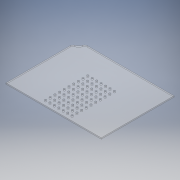
# Autodesk Inventor part: Plaque inferieur
Saved by Autodesk Inventor 2017 (Build 210142000, 142)
## iProperties
Company: FABLAB Frenchmakers
Part Number: Plaque inferieur
Project: 1400-PopCorn Machine
Material: Plastique PMMA
Catalog Web Link: http://www.frenchmakers.com/
Document SubType Name: Modeling
Designer: FABLAB Frenchmakers
Density: 1.188 g/cm^3
Appearance: Polycarbonate - Transparent
Stock Number: 1400-04-01
Author: Adrien MARY
Autodesk Inventor part; units mm, degrees
ref_plane "YZ Plane" through (0, 0, 0) normal (1, 0, 0) x (0, 1, 0)
ref_plane "XZ Plane" through (0, 0, 0) normal (0, 1, 0) x (-1, 0, 0)
ref_plane "XY Plane" through (0, 0, 0) normal (0, 0, 1) x (1, 0, 0)
sketch "Esquisse1" plane through (0, 0, 0) normal (0, 0, 1) x (1, 0, 0)
  line L0 (-192.7, -147.2) -> (192.7, -147.2)
  line L1 (192.7, -147.2) -> (192.7, 147.2)
  line L2 (192.7, 147.2) -> (-192.7, 147.2)
  line L3 (-192.7, 147.2) -> (-192.7, -147.2)
  line L4 (-192.7, -147.2) -> (192.7, 147.2) construction
  line L5 (192.7, -147.2) -> (-192.7, 147.2) construction
  point P0 (0, 0)
  dimension "Largueur_plaque_inf" = 385.4
  dimension "Profondeur_plaque_inf" = 294.4
  constraints: 12 end point, 2 midpoint, 2 parallel, 1 horizontal, 1 perpendicular
  measures "Largueur_plaque_inf" distance of L1.end L2.end
  measures "Profondeur_plaque_inf" distance of L2.end L0.start
extrude "Embase" add sketch "Esquisse1" along normal mid plane 5
sketch "Esquisse2" plane through (0, 0, 2.5) normal (0, 0, 1) x (1, 0, 0)
  point P0 (0, 0)
  point P1 (-53, -127)
  dimension "d4" = 53
  dimension "d5" = 127
  measures "d4" horizontal distance of point (0, 0) point (-53, -127)
  measures "d5" vertical distance of point (0, 0) point (-53, -127)
hole "Perçage" at (-53, -127, 2.5) direction (0, 0, -1) diameter 7.5 end through all
pattern_linear "Réseau rectangulaire largueur" count 7 spacing 18 along (1, 0, 0) of "Perçage"
pattern_linear "Réseau rectangulaire profondeur" count 10 spacing 19 along (0, 1, 0) of "Perçage", "Réseau rectangulaire largueur"
sketch "Esquisse3" plane through (0, 0, 2.5) normal (0, 0, 1) x (1, 0, 0)
  circle A0 centre (-192.7, 147.2) radius 25
  line L0 (192.7, 147.2) -> (-192.7, 147.2) construction
  line L1 (-192.7, 147.2) -> (-192.7, -147.2) construction
  point P0 (0, 0)
  dimension "d19" = 50
  constraints: 1 centre point, 1 coincident
  measures "d19" diameter of A0
extrude "Passage cable" cut sketch "Esquisse3" against normal through all
fillet "Congé1" radius 10 2 edges at (-192.7, 122.2, 0) (-167.7, 147.2, 0)
